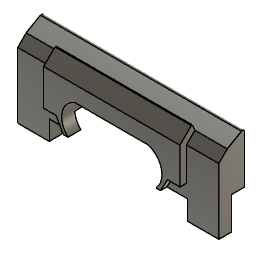
GBM v13 (Autodesk Fusion 360 design; units mm, degrees)
Autodesk Fusion 360 part; units mm, degrees
sketch "Boceto1" plane through (0, 0, 0) normal (0, 1, 0) x (1, 0, 0)
  line L0 (-6.315, -4.3) -> (6.315, -4.3)
  line L1 (6.315, -4.3) -> (6.315, 0)
  line L2 (6.315, 0) -> (-6.315, 0)
  line L3 (-6.315, 0) -> (-6.315, -4.3)
  line L4 (-6.315, -3.25) -> (6.315, -3.25)
  line L5 (-4.5, 1.2) -> (4.5, 1.2)
  line L6 (-5.165, 0) -> (-4.5, 1.2)
  line L7 (5.165, 0) -> (4.5, 1.2)
  point P0 (-5.165, 0)
  point P1 (5.165, 0)
  dimension "d1" = 12.63
  dimension "d2" = 6.315
  dimension "d3" = 4.3
  dimension "d4" = 3.25
  dimension "d5" = 1.15
  dimension "d6" = 1.15
  dimension "d7" = 9
  dimension "d8" = 4.5
  dimension "d15" = 1.05
  dimension "d45" = 1.2
  constraint horizontal L0
  constraint vertical L1
  constraint horizontal L2
  constraint vertical L3
  constraint coincident L3 L4.start
  constraint coincident L1 L4.end
  constraint perpendicular L1 L4
  constraint coincident L2 P0
  constraint coincident L2 P1
  constraint horizontal L5
  constraint coincident P0 L6.start
  constraint coincident P1 L7.start
  measures "d1" distance of L0.start L0.end
  measures "d2" horizontal distance of origin L0.start
  measures "d3" distance of L0.start L2.end
  measures "d4" distance of L2.end L4.start
  measures "d5" distance of L2.end P0
  measures "d6" distance of L1.end P1
  measures "d7" distance of L5.start L5.end
  measures "d8" horizontal distance of origin L5.start
  measures "d15" distance of L0.start L4.start
  measures "d45" vertical distance of L2.end L5.start
extrude "Extruir1" add sketch "Boceto1" along normal blind 0.6 contours L2 L5 L6 L7
extrude "Extruir2" add sketch "Boceto1" along normal blind 3 contours L0 L1 L3 L4 | L1 L2 L3 L4
extrude "Extruir9" add 1 faces at (-2.105, 1, 4.3) along direction (0, 0, 1) blind 0.1
chamfer "Chaflán3" distance 1.05 angle 45 1 edges at (0, 0, 4.4)
sketch "Boceto2" plane through (-6.315, 0, 0) normal (-1, 0, 0) x (0, -1, 0)
  line L0 (-3, 4.4) -> (-3, 0)
  line L1 (-3, 0) -> (0, 0)
  line L2 (0, 0) -> (0, 3.35)
  line L3 (-0.6, 3.85) -> (-0.6, 0)
  line L4 (-3, 3.8) -> (-0.45, 3.8)
  line L5 (-1.15, 4.4) -> (-2.8988, 4.4) construction
  line L6 (-1.52, 3.8) -> (-2.8897, 3.8) construction
  line L7 (-1.3829, 3.8594) -> (-2.3193, 4.4)
  line L8 (-1.3829, 3.8594) -> (-1.9443, 3.8594) construction
  line L9 (-2.3193, 4.4) -> (-3, 4.793)
  line L10 (-3, 4.4) -> (-3, 4.793)
  line L11 (0, 3.35) -> (-1.05, 4.4)
  line L12 (-1.05, 4.4) -> (-3, 4.4)
  line L13 (-1.3829, 3.8594) -> (-1.15, 4.4)
  line L14 (-1.3829, 3.8594) -> (-0.6, 3.0765)
  line L15 (-1.3829, 3.8594) -> (-0.2757, 3.8594) construction
  dimension "d20" = 0.6
  dimension "d31" = 0.6
  dimension "d37" = 30
  dimension "d50" = 45
  constraint perpendicular L1 L3
  constraint horizontal L4
  constraint coincident L1 L3.end
  constraint coincident L0 L4.start
  constraint horizontal L5
  constraint horizontal L6
  constraint coincident L4 L6.start
  constraint horizontal L8
  constraint coincident L5 L7.end
  constraint parallel L7 L9
  constraint coincident L0.start L10.start
  constraint horizontal L15
  constraint coincident L3 L14.end
  measures "d20" distance of L0.start L4.start
  measures "d31" distance of L1.end L3.end
  measures "d37" angle of L7 L8
  measures "d50" angle of L14 L15
extrude "Extruir4" add sketch "Boceto2" against normal blind 15.63 contours L0 L1 L3 L4 L14
extrude "Extruir3" add sketch "Boceto2" along normal blind 3 contours L0 L1 L3 L4 L14
sketch "Boceto3" plane through (0, 0, 0) normal (0, 0, -1) x (1, 0, 0)
  line L0 (6.315, -0.6) -> (6.315, 0)
  line L1 (6.315, 0) -> (5.165, 0)
  line L2 (5.165, 0) -> (5.165, -0.6)
  line L3 (5.165, -0.6) -> (-5.165, -0.6)
  line L4 (-5.165, -0.6) -> (-5.165, 0)
  line L5 (-5.165, 0) -> (-6.315, 0)
  line L6 (-6.315, 0) -> (-6.315, -0.6)
  line L7 (-6.315, -0.6) -> (-9.315, -0.6)
  line L8 (-9.315, -0.6) -> (-9.315, -3)
  line L9 (-9.315, -3) -> (9.315, -3)
  line L10 (9.315, -3) -> (9.315, -0.6)
  line L11 (9.315, -0.6) -> (6.315, -0.6)
  line L12 (-6.4, -0.6) -> (-6.4, -3)
  line L13 (6.4, -0.6) -> (6.4, -3)
  line L14 (-9.315, -1.8) -> (9.315, -1.8)
  dimension "d25" = 6.4
  dimension "d26" = 6.4
  dimension "d27" = 1.2
  constraint coincident L7 L12.start
  constraint coincident L9 L12.end
  constraint perpendicular L9 L12
  constraint coincident L11 L13.start
  constraint coincident L9 L13.end
  constraint perpendicular L9 L13
  constraint coincident L8 L14.start
  constraint coincident L10 L14.end
  constraint perpendicular L10 L14
  measures "d25" horizontal distance of origin L12.start
  measures "d26" horizontal distance of origin L13.start
  measures "d27" distance of L7.end L14.start
extrude "Extruir5" add sketch "Boceto3" along normal blind 3 contours L10 L11 L13 L14 | L7 L8 L12 L14
extrude "Extruir7" cut sketch "Boceto2" against normal blind 20 contours L7 L12 L13
extrude "Extruir8" add sketch "Boceto2" against normal blind 12.63 contours L9 L10 L12
extrude "Extruir11" add sketch "Boceto2" against normal blind 15.63 contours L0 L4 L7 L12 L14 | L9 L10 L12
extrude "Extruir10" add sketch "Boceto2" along normal blind 3 contours L0 L4 L7 L12 L14 | L9 L10 L12
fillet "Empalme1" radius 0.2 1 edges at (0, 3, 4.793)
sketch "Boceto4" plane through (0, 0, 0) normal (0, -1, 0) x (1, 0, 0)
  line L0 (6.315, 3.35) -> (-6.315, 3.35)
  line L1 (-6.315, 3.35) -> (-6.315, 0)
  line L2 (-6.315, 0) -> (-5.165, 0)
  line L3 (-5.165, 0) -> (-4.5, -1.2)
  line L4 (-4.5, -1.2) -> (4.5, -1.2)
  line L5 (4.5, -1.2) -> (5.165, 0)
  line L6 (5.165, 0) -> (6.315, 0)
  line L7 (6.315, 0) -> (6.315, 3.35)
  line L8 (-4.65, 3.35) -> (-4.65, -1.2)
  line L9 (4.65, 3.35) -> (4.65, -1.2)
  line L10 (-4.65, 0.15) -> (4.65, 0.15)
  line L11 (-3.4, -1.6) -> (3.4, -1.6)
  arc A0 (-3.4, 1.9) -> (-3.4, -1.6) centre (-2.8, 0.15) ccw
  arc A1 (3.4, -1.6) -> (3.4, 1.9) centre (2.8, 0.15) ccw
  line L12 (-3.4, 1.9) -> (-3.4, -1.6)
  line L13 (3.4, 1.9) -> (3.4, -1.6)
  line L14 (-3.4, 1.9) -> (3.4, 1.9)
  point P0 (-3.4, -1.6)
  point P1 (3.4, -1.6)
  dimension "d55" = 4.65
  dimension "d56" = 4.65
  dimension "d59" = 3.4
  dimension "d60" = 3.4
  dimension "d67" = 0.4
  dimension "d68" = 0.4
  dimension "d70" = 3.5
  dimension "d71" = 1.75
  constraint coincident L0 L8.start
  constraint coincident L4 L8.end
  constraint perpendicular L4 L8
  constraint coincident L0 L9.start
  constraint coincident L4 L9.end
  constraint perpendicular L4 L9
  constraint coincident L8 L10.start
  constraint coincident L9 L10.end
  constraint perpendicular L9 L10
  constraint coincident P0 L11.start
  constraint coincident P1 L11.end
  constraint coincident L10.start A0
  constraint coincident L10.end A1
  constraint horizontal L14
  measures "d55" horizontal distance of origin L8.start
  measures "d56" horizontal distance of origin L9.start
  measures "d59" horizontal distance of origin A0.start
  measures "d60" horizontal distance of origin A1.end
  measures "d67" vertical distance of L3.end P0
  measures "d68" vertical distance of L4.end P1
  measures "d70" distance of A1.end P1
  measures "d71" vertical distance of L10.end P1
extrude "Extruir12" cut sketch "Boceto4" against normal blind 5 contours L4 L10 A1 L13 | L10 A1 L13 | L10 A0 L12 | L4 L10 A0 L12 | L4 L10 L12 L13 | L10 L12 L13 L14
sketch "Boceto5" plane through (0, 0, 0) normal (0, 0, -1) x (1, 0, 0)
  line L0 (-4.6439, -0.6) -> (-5.165, -0.6)
  line L1 (-5.165, -0.6) -> (-5.165, 0)
  line L2 (-5.165, 0) -> (-6.315, 0)
  line L3 (-6.315, 0) -> (-6.315, -0.6)
  line L4 (-6.315, -0.6) -> (-6.4, -0.6)
  line L5 (-6.4, -0.6) -> (-6.4, -1.8)
  line L6 (-6.4, -1.8) -> (-9.315, -1.8)
  line L7 (-9.315, -1.8) -> (-9.315, -3)
  line L8 (-9.315, -3) -> (-4.6439, -3)
  line L9 (9.315, -3) -> (9.315, -1.8)
  line L10 (9.315, -1.8) -> (6.4, -1.8)
  line L11 (6.4, -1.8) -> (6.4, -0.6)
  line L12 (6.4, -0.6) -> (6.315, -0.6)
  line L13 (6.315, -0.6) -> (6.315, 0)
  line L14 (6.315, 0) -> (5.165, 0)
  line L15 (5.165, 0) -> (5.165, -0.6)
  line L16 (-6.315, -0.6) -> (-5.165, -0.6)
  line L17 (5.165, -0.6) -> (6.315, -0.6)
  line L18 (-4.1, -0.6) -> (-4.1, -1.2)
  line L19 (4.1, -0.6) -> (4.1, -1.2)
  line L20 (-6.4, -1.2) -> (-4.1, -1.2)
  line L21 (4.1, -1.2) -> (6.4, -1.2)
  line L22 (-4.6439, -3) -> (-4.6439, -0.6)
  line L23 (4.6439, -0.6) -> (4.6439, -3)
  line L24 (4.6439, -3) -> (9.315, -3)
  line L25 (5.165, -0.6) -> (4.6439, -0.6)
  line L26 (-4.1, -0.6) -> (-5.165, -0.6)
  line L27 (4.1, -0.6) -> (4.6439, -0.6)
  dimension "d16" = 0.6
  dimension "d18" = 0.82
  dimension "d57" = 3.5
  dimension "d63" = 2.3
  dimension "d64" = 2.3
  dimension "d72" = 0.6
  constraint coincident L3.end L4.start
  constraint coincident L0.end L1.start
  constraint coincident L15.end L17.start
  constraint coincident L12.end L13.start
  constraint coincident L5 L20.start
  constraint coincident L11 L21.end
  constraint perpendicular L11 L20
  constraint coincident L0 L18.start
  constraint perpendicular L18 L20
  constraint coincident L17 L19.start
  constraint coincident L19.end L20
  constraint perpendicular L19 L20
  constraint collinear L20 L21
  constraint coincident L23.start L25.end
  measures "d63" distance of L20.start L18.end
  measures "d64" distance of L21.end L19.end
  measures "d72" distance of L19.start L19.end
extrude "Extruir13" add sketch "Boceto5" along normal blind 1.2 contours L0 L4 L5 L16 L20 L22 L26 | L11 L12 L17 L21 L23 L25
extrude "Extruir14" add 2 faces at (4.4644, 0.6, -1.0467) (-4.4644, 0.6, -1.0467) along direction (0, 1, 0) blind 0.6
extrude "Extruir15" add 1 faces at (4.6439, 0.8, -1.0269) along direction (-1, 0, 0) blind 0.2
extrude "Extruir16" add 1 faces at (-4.6439, 1, -1.0269) along direction (1, 0, 0) blind 0.2
equation "d2 = d1 / 2"
equation "d6 = d5"
equation "d8 = d7 / 2"
equation "d20 = d16"
equation "d23 = -d1 - 3 mm"
equation "d26 = d25"
equation "d40 = -d1"
equation "d48 = d15"
equation "d53 = -12.63 mm - 3 mm"
equation "d56 = d55"
equation "d60 = d59"
equation "d64 = d63"
equation "d68 = d67"
equation "d71 = d70 / 2"
